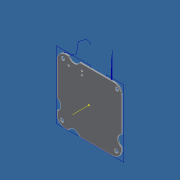
# Autodesk Inventor part: Eagle PCB
Saved by Autodesk Inventor 2016 (Build 200138000, 138)
## iProperties
Created: 2015-06-19
Part Number: Eagle PCB
Material: Generic
Document SubType Name: Modeling
Designer: Samuel Clay
Density: 1 g/cm^3
Appearance: Default
Author: Samuel Clay
Autodesk Inventor part; units mm, degrees
(part 1 of 11)
ref_plane "YZ Plane" through (0, 0, 0) normal (1, 0, 0) x (0, 1, 0)
ref_plane "XZ Plane" through (0, 0, 0) normal (0, 1, 0) x (-1, 0, 0)
ref_plane "XY Plane" through (0, 0, 0) normal (0, 0, 1) x (1, 0, 0)
sketch "1" plane through (0, 0, 0) normal (0, 0, 1) x (1, 0, 0)
  arc A0 (13.5069, 27.1331) -> (13.4171, 27.2229) centre (13.462, 27.178) ccw
  arc A1 (12.9091, 26.7149) -> (12.9989, 26.6251) centre (12.954, 26.67) ccw
  line L0 (13.462, 27.178) -> (12.954, 26.67)
  arc A2 (14.6362, 27.1145) -> (14.6362, 27.2415) centre (14.6362, 27.178) ccw
  arc A3 (13.462, 27.2415) -> (13.462, 27.1145) centre (13.462, 27.178) ccw
  line L1 (14.6362, 27.178) -> (13.462, 27.178)
  arc A4 (3.5302, 16.6256) -> (3.4404, 16.5358) centre (3.4853, 16.5807) ccw
  arc A5 (10.6231, 9.3531) -> (10.7129, 9.4429) centre (10.668, 9.398) ccw
  line L2 (3.4853, 16.5807) -> (10.668, 9.398)
  arc A6 (3.5488, 24.0433) -> (3.4218, 24.0433) centre (3.4853, 24.0433) ccw
  arc A7 (3.4218, 16.5807) -> (3.5488, 16.5807) centre (3.4853, 16.5807) ccw
  line L3 (3.4853, 24.0433) -> (3.4853, 16.5807)
  arc A8 (20.2591, 27.3871) -> (20.3489, 27.4769) centre (20.304, 27.432) ccw
  arc A9 (17.5549, 30.2709) -> (17.4651, 30.1811) centre (17.51, 30.226) ccw
  line L4 (20.304, 27.432) -> (17.51, 30.226)
  arc A10 (26.162, 27.3685) -> (26.162, 27.4955) centre (26.162, 27.432) ccw
  arc A11 (20.304, 27.4955) -> (20.304, 27.3685) centre (20.304, 27.432) ccw
  line L5 (26.162, 27.432) -> (20.304, 27.432)
  arc A12 (17.5549, 30.0069) -> (17.4651, 30.0967) centre (17.51, 30.0518) ccw
  arc A13 (15.3142, 27.9458) -> (15.404, 27.856) centre (15.3591, 27.9009) ccw
  line L6 (17.51, 30.0518) -> (15.3591, 27.9009)
  arc A14 (17.5735, 30.226) -> (17.4465, 30.226) centre (17.51, 30.226) ccw
  arc A15 (17.4465, 30.0518) -> (17.5735, 30.0518) centre (17.51, 30.0518) ccw
  line L7 (17.51, 30.226) -> (17.51, 30.0518)
  arc A16 (17.5735, 35.052) -> (17.4465, 35.052) centre (17.51, 35.052) ccw
  arc A17 (17.4465, 30.226) -> (17.5735, 30.226) centre (17.51, 30.226) ccw
  line L8 (17.51, 35.052) -> (17.51, 30.226)
  arc A18 (8.1889, 27.4609) -> (8.0991, 27.3711) centre (8.144, 27.416) ccw
  arc A19 (9.3531, 26.1171) -> (9.4429, 26.2069) centre (9.398, 26.162) ccw
  line L9 (8.144, 27.416) -> (9.398, 26.162)
  arc A20 (8.2075, 28.702) -> (8.0805, 28.702) centre (8.144, 28.702) ccw
  arc A21 (8.0805, 27.416) -> (8.2075, 27.416) centre (8.144, 27.416) ccw
  line L10 (8.144, 28.702) -> (8.144, 27.416)
  arc A22 (26.1171, 31.6777) -> (26.2069, 31.5879) centre (26.162, 31.6328) ccw
  arc A23 (27.4601, 32.8411) -> (27.3704, 32.9309) centre (27.4152, 32.886) ccw
  line L11 (26.162, 31.6328) -> (27.4153, 32.886)
  arc A24 (26.0985, 27.432) -> (26.2255, 27.432) centre (26.162, 27.432) ccw
  arc A25 (26.2255, 31.6328) -> (26.0985, 31.6328) centre (26.162, 31.6328) ccw
  line L12 (26.162, 27.432) -> (26.162, 31.6328)
  arc A26 (26.2069, 24.1749) -> (26.1171, 24.0851) centre (26.162, 24.13) ccw
  arc A27 (26.8791, 23.3231) -> (26.9689, 23.4129) centre (26.924, 23.368) ccw
  line L13 (26.162, 24.13) -> (26.924, 23.368)
  arc A28 (26.2255, 27.432) -> (26.0985, 27.432) centre (26.162, 27.432) ccw
  arc A29 (26.0985, 24.13) -> (26.2255, 24.13) centre (26.162, 24.13) ccw
  line L14 (26.162, 27.432) -> (26.162, 24.13)
  arc A30 (33.8827, 24.1749) -> (33.7929, 24.0851) centre (33.8378, 24.13) ccw
  arc A31 (34.8303, 23.0477) -> (34.9201, 23.1375) centre (34.8752, 23.0926) ccw
  line L15 (33.8378, 24.13) -> (34.8752, 23.0926)
  arc A32 (32.258, 24.1935) -> (32.258, 24.0665) centre (32.258, 24.13) ccw
  arc A33 (33.8378, 24.0665) -> (33.8378, 24.1935) centre (33.8378, 24.13) ccw
  line L16 (32.258, 24.13) -> (33.8378, 24.13)
  arc A34 (31.4511, 23.4129) -> (31.5409, 23.3231) centre (31.496, 23.368) ccw
  arc A35 (32.3029, 24.0851) -> (32.2131, 24.1749) centre (32.258, 24.13) ccw
  line L17 (31.496, 23.368) -> (32.258, 24.13)
  arc A36 (26.924, 23.4315) -> (26.924, 23.3045) centre (26.924, 23.368) ccw
  arc A37 (31.496, 23.3045) -> (31.496, 23.4315) centre (31.496, 23.368) ccw
  line L18 (26.924, 23.368) -> (31.496, 23.368)
  arc A38 (23.4571, 19.9909) -> (23.5469, 19.9011) centre (23.502, 19.946) ccw
  arc A39 (26.9689, 23.3231) -> (26.8791, 23.4129) centre (26.924, 23.368) ccw
  line L19 (23.502, 19.946) -> (26.924, 23.368)
  arc A40 (23.314, 20.0095) -> (23.314, 19.8825) centre (23.314, 19.946) ccw
  arc A41 (23.502, 19.8825) -> (23.502, 20.0095) centre (23.502, 19.946) ccw
  line L20 (23.314, 19.946) -> (23.502, 19.946)
  arc A42 (29.7389, 12.8851) -> (29.6491, 12.9749) centre (29.694, 12.93) ccw
  arc A43 (27.3871, 10.7129) -> (27.4769, 10.6231) centre (27.432, 10.668) ccw
  line L21 (29.694, 12.93) -> (27.432, 10.668)
  arc A44 (31.242, 12.8665) -> (31.242, 12.9935) centre (31.242, 12.93) ccw
  arc A45 (29.694, 12.9935) -> (29.694, 12.8665) centre (29.694, 12.93) ccw
  line L22 (31.242, 12.93) -> (29.694, 12.93)
  arc A46 (36.0231, 21.8549) -> (36.1129, 21.9447) centre (36.068, 21.8998) ccw
  arc A47 (34.9201, 23.1375) -> (34.8303, 23.0477) centre (34.8752, 23.0926) ccw
  line L23 (36.068, 21.8998) -> (34.8752, 23.0926)
  arc A48 (36.0045, 14.986) -> (36.1315, 14.986) centre (36.068, 14.986) ccw
  arc A49 (36.1315, 21.8998) -> (36.0045, 21.8998) centre (36.068, 21.8998) ccw
  line L24 (36.068, 14.986) -> (36.068, 21.8998)
  arc A50 (33.9671, 12.9749) -> (34.0569, 12.8851) centre (34.012, 12.93) ccw
  arc A51 (36.1129, 14.9411) -> (36.0231, 15.0309) centre (36.068, 14.986) ccw
  line L25 (34.012, 12.93) -> (36.068, 14.986)
  arc A52 (31.242, 12.9935) -> (31.242, 12.8665) centre (31.242, 12.93) ccw
  arc A53 (34.012, 12.8665) -> (34.012, 12.9935) centre (34.012, 12.93) ccw
  line L26 (31.242, 12.93) -> (34.012, 12.93)
  arc A54 (15.5549, 28.0069) -> (15.4651, 28.0967) centre (15.51, 28.0518) ccw
  arc A55 (15.3142, 27.9458) -> (15.404, 27.856) centre (15.3591, 27.9009) ccw
  line L27 (15.51, 28.0518) -> (15.3591, 27.9009)
  arc A56 (14.5913, 27.2229) -> (14.6811, 27.1331) centre (14.6362, 27.178) ccw
  arc A57 (15.404, 27.856) -> (15.3142, 27.9458) centre (15.3591, 27.9009) ccw
  line L28 (14.6362, 27.178) -> (15.3591, 27.9009)
  arc A58 (7.9362, 30.0011) -> (7.8118, 29.9749) centre (7.874, 29.988) ccw
  arc A59 (8.0818, 28.6889) -> (8.2062, 28.7151) centre (8.144, 28.702) ccw
  line L29 (7.874, 29.988) -> (8.144, 28.702)
  arc A60 (7.9375, 31.623) -> (7.8105, 31.623) centre (7.874, 31.623) ccw
  arc A61 (7.8105, 29.988) -> (7.9375, 29.988) centre (7.874, 29.988) ccw
  line L30 (7.874, 31.623) -> (7.874, 29.988)
  arc A62 (3.4404, 24.0882) -> (3.5302, 23.9984) centre (3.4853, 24.0433) ccw
  arc A63 (8.1889, 28.6571) -> (8.0991, 28.7469) centre (8.144, 28.702) ccw
  line L31 (3.4853, 24.0433) -> (8.144, 28.702)
  arc A64 (3.3727, 24.1068) -> (3.3727, 23.9798) centre (3.3727, 24.0433) ccw
  arc A65 (3.4853, 23.9798) -> (3.4853, 24.1068) centre (3.4853, 24.0433) ccw
  line L32 (3.3727, 24.0433) -> (3.4853, 24.0433)
  arc A66 (-1.8796, -1.524) -> (-1.6764, -1.524) centre (-1.778, -1.524) ccw
  arc A67 (-1.6764, 38.608) -> (-1.8796, 38.608) centre (-1.778, 38.608) ccw
  line L33 (-1.778, -1.524) -> (-1.778, 38.608)
  arc A68 (38.354, -1.6256) -> (38.354, -1.4224) centre (38.354, -1.524) ccw
  arc A69 (-1.778, -1.4224) -> (-1.778, -1.6256) centre (-1.778, -1.524) ccw
  line L34 (38.354, -1.524) -> (-1.778, -1.524)
  arc A70 (38.2016, 38.6086) -> (37.9984, 38.6074) centre (38.1, 38.608) ccw
  arc A71 (38.2524, -1.5246) -> (38.4556, -1.5234) centre (38.354, -1.524) ccw
  line L35 (38.1, 38.608) -> (38.354, -1.524)
  arc A72 (27.94, 38.7096) -> (27.94, 38.5064) centre (27.94, 38.608) ccw
  arc A73 (38.1, 38.5064) -> (38.1, 38.7096) centre (38.1, 38.608) ccw
  line L36 (27.94, 38.608) -> (38.1, 38.608)
  arc A74 (27.8384, 34.036) -> (28.0416, 34.036) centre (27.94, 34.036) ccw
  arc A75 (28.0416, 38.608) -> (27.8384, 38.608) centre (27.94, 38.608) ccw
  line L37 (27.94, 34.036) -> (27.94, 38.608)
  arc A76 (25.654, 34.1376) -> (25.654, 33.9344) centre (25.654, 34.036) ccw
  arc A77 (27.94, 33.9344) -> (27.94, 34.1376) centre (27.94, 34.036) ccw
  line L38 (25.654, 34.036) -> (27.94, 34.036)
  arc A78 (21.2642, 29.7898) -> (21.4078, 29.6462) centre (21.336, 29.718) ccw
  arc A79 (25.7258, 33.9642) -> (25.5822, 34.1078) centre (25.654, 34.036) ccw
  line L39 (21.336, 29.718) -> (25.654, 34.036)
  arc A80 (18.6104, 32.3332) -> (18.4736, 32.1828) centre (18.542, 32.258) ccw
  arc A81 (21.2676, 29.6428) -> (21.4044, 29.7932) centre (21.336, 29.718) ccw
  line L40 (18.542, 32.258) -> (21.336, 29.718)
  arc A82 (18.6436, 38.608) -> (18.4404, 38.608) centre (18.542, 38.608) ccw
  arc A83 (18.4404, 32.258) -> (18.6436, 32.258) centre (18.542, 32.258) ccw
  line L41 (18.542, 38.608) -> (18.542, 32.258)
  arc A84 (-1.778, 38.7096) -> (-1.778, 38.5064) centre (-1.778, 38.608) ccw
  arc A85 (18.542, 38.5064) -> (18.542, 38.7096) centre (18.542, 38.608) ccw
  line L42 (-1.778, 38.608) -> (18.542, 38.608)
  arc A86 (16.256, 16.4465) -> (16.256, 16.5735) centre (16.256, 16.51) ccw
  arc A87 (14.732, 16.5735) -> (14.732, 16.4465) centre (14.732, 16.51) ccw
  line L43 (16.256, 16.51) -> (14.732, 16.51)
  arc A88 (21.5046, 21.6688) -> (21.4148, 21.7586) centre (21.4597, 21.7137) ccw
  arc A89 (16.2111, 16.5549) -> (16.3009, 16.4651) centre (16.256, 16.51) ccw
  line L44 (21.4597, 21.7137) -> (16.256, 16.51)
  arc A90 (21.5463, 21.6502) -> (21.5463, 21.7772) centre (21.5463, 21.7137) ccw
  arc A91 (21.4597, 21.7772) -> (21.4597, 21.6503) centre (21.4597, 21.7137) ccw
  line L45 (21.5463, 21.7137) -> (21.4597, 21.7137)
  arc A92 (34.5889, 16.4651) -> (34.4991, 16.5549) centre (34.544, 16.51) ccw
  arc A93 (34.2451, 16.3009) -> (34.3349, 16.2111) centre (34.29, 16.256) ccw
  line L46 (34.544, 16.51) -> (34.29, 16.256)
  arc A94 (34.6075, 19.812) -> (34.4805, 19.812) centre (34.544, 19.812) ccw
  arc A95 (34.4805, 16.51) -> (34.6075, 16.51) centre (34.544, 16.51) ccw
  line L47 (34.544, 19.812) -> (34.544, 16.51)
  arc A96 (33.1524, 21.2934) -> (33.0626, 21.2036) centre (33.1075, 21.2485) ccw
  arc A97 (34.4991, 19.7671) -> (34.5889, 19.8569) centre (34.544, 19.812) ccw
  line L48 (33.1075, 21.2485) -> (34.544, 19.812)
  arc A98 (33.171, 21.3248) -> (33.044, 21.3248) centre (33.1075, 21.3248) ccw
  arc A99 (33.044, 21.2485) -> (33.171, 21.2485) centre (33.1075, 21.2485) ccw
  line L49 (33.1075, 21.3248) -> (33.1075, 21.2485)
  arc A100 (35.7691, 27.8951) -> (35.8589, 27.9849) centre (35.814, 27.94) ccw
  arc A101 (35.6049, 28.2389) -> (35.5151, 28.1491) centre (35.56, 28.194) ccw
  line L50 (35.814, 27.94) -> (35.56, 28.194)
  arc A102 (35.7505, 27.432) -> (35.8775, 27.432) centre (35.814, 27.432) ccw
  arc A103 (35.8775, 27.94) -> (35.7505, 27.94) centre (35.814, 27.94) ccw
  line L51 (35.814, 27.432) -> (35.814, 27.94)
  arc A104 (34.4414, 26.1492) -> (34.5312, 26.0594) centre (34.4863, 26.1043) ccw
  arc A105 (35.8589, 27.3871) -> (35.7691, 27.4769) centre (35.814, 27.432) ccw
  line L52 (34.4863, 26.1043) -> (35.814, 27.432)
  arc A106 (34.4228, 25.815) -> (34.5498, 25.815) centre (34.4863, 25.815) ccw
  arc A107 (34.5498, 26.1043) -> (34.4228, 26.1043) centre (34.4863, 26.1043) ccw
  line L53 (34.4863, 25.815) -> (34.4863, 26.1043)
  arc A108 (21.1269, 15.7031) -> (21.0371, 15.7929) centre (21.082, 15.748) ccw
  arc A109 (20.7831, 15.5389) -> (20.8729, 15.4491) centre (20.828, 15.494) ccw
  line L54 (21.082, 15.748) -> (20.828, 15.494)
  arc A110 (24.384, 15.6845) -> (24.384, 15.8115) centre (24.384, 15.748) ccw
  arc A111 (21.082, 15.8115) -> (21.082, 15.6845) centre (21.082, 15.748) ccw
  line L55 (24.384, 15.748) -> (21.082, 15.748)
  arc A112 (25.9752, 17.2494) -> (25.8854, 17.3392) centre (25.9303, 17.2943) ccw
  arc A113 (24.3391, 15.7929) -> (24.4289, 15.7031) centre (24.384, 15.748) ccw
  line L56 (25.9303, 17.2943) -> (24.384, 15.748)
  arc A114 (25.9657, 17.2308) -> (25.9657, 17.3578) centre (25.9657, 17.2943) ccw
  arc A115 (25.9303, 17.3578) -> (25.9303, 17.2308) centre (25.9303, 17.2943) ccw
  line L57 (25.9657, 17.2943) -> (25.9303, 17.2943)
  arc A116 (30.022, 30.3658) -> (30.1118, 30.276) centre (30.0669, 30.3209) ccw
  arc A117 (32.5569, 32.7211) -> (32.4671, 32.8109) centre (32.512, 32.766) ccw
  line L58 (30.0669, 30.3209) -> (32.512, 32.766)
  arc A118 (30.0034, 30.2344) -> (30.1304, 30.2344) centre (30.0669, 30.2344) ccw
  arc A119 (30.1304, 30.3209) -> (30.0034, 30.3209) centre (30.0669, 30.3209) ccw
  line L59 (30.0669, 30.2344) -> (30.0669, 30.3209)
  arc A120 (9.3345, 19.304) -> (9.4615, 19.304) centre (9.398, 19.304) ccw
  arc A121 (9.4615, 20.32) -> (9.3345, 20.32) centre (9.398, 20.32) ccw
  line L60 (9.398, 19.304) -> (9.398, 20.32)
  arc A122 (13.9251, 14.6871) -> (14.0149, 14.7769) centre (13.97, 14.732) ccw
  arc A123 (9.4429, 19.3489) -> (9.3531, 19.2591) centre (9.398, 19.304) ccw
  line L61 (13.97, 14.732) -> (9.398, 19.304)
  arc A124 (27.432, 14.6685) -> (27.432, 14.7955) centre (27.432, 14.732) ccw
  arc A125 (13.97, 14.7955) -> (13.97, 14.6685) centre (13.97, 14.732) ccw
  line L62 (27.432, 14.732) -> (13.97, 14.732)
  arc A126 (28.7329, 15.9431) -> (28.6431, 16.0329) centre (28.688, 15.988) ccw
  arc A127 (27.3871, 14.7769) -> (27.4769, 14.6871) centre (27.432, 14.732) ccw
  line L63 (28.6881, 15.9881) -> (27.432, 14.732)
  arc A128 (28.7516, 16.9054) -> (28.6246, 16.9054) centre (28.6881, 16.9054) ccw
  arc A129 (28.6246, 15.9881) -> (28.7515, 15.9881) centre (28.6881, 15.9881) ccw
  line L64 (28.6881, 16.9054) -> (28.6881, 15.9881)
  arc A130 (29.1405, 31.2622) -> (29.2255, 31.1678) centre (29.183, 31.215) ccw
  arc A131 (31.7925, 33.4808) -> (31.7075, 33.5752) centre (31.75, 33.528) ccw
  line L65 (29.183, 31.215) -> (31.75, 33.528)
  arc A132 (29.1195, 31.1183) -> (29.2465, 31.1183) centre (29.183, 31.1183) ccw
  arc A133 (29.2465, 31.215) -> (29.1195, 31.215) centre (29.183, 31.215) ccw
  line L66 (29.183, 31.1183) -> (29.183, 31.215)
  arc A134 (31.9591, 16.3009) -> (32.0489, 16.2111) centre (32.004, 16.256) ccw
  arc A135 (33.5729, 17.7351) -> (33.4831, 17.8249) centre (33.528, 17.78) ccw
  line L67 (32.004, 16.256) -> (33.528, 17.78)
  arc A136 (31.242, 16.3195) -> (31.242, 16.1925) centre (31.242, 16.256) ccw
  arc A137 (32.004, 16.1925) -> (32.004, 16.3195) centre (32.004, 16.256) ccw
  line L68 (31.242, 16.256) -> (32.004, 16.256)
  arc A138 (29.7536, 17.8342) -> (29.6638, 17.7444) centre (29.7087, 17.7893) ccw
  arc A139 (31.1971, 16.2111) -> (31.2869, 16.3009) centre (31.242, 16.256) ccw
  line L69 (29.7087, 17.7893) -> (31.242, 16.256)
  arc A140 (29.5719, 17.8528) -> (29.5719, 17.7258) centre (29.5719, 17.7893) ccw
  arc A141 (29.7087, 17.7258) -> (29.7087, 17.8528) centre (29.7087, 17.7893) ccw
  line L70 (29.5719, 17.7893) -> (29.7087, 17.7893)
  arc A142 (12.291, 17.7883) -> (12.2011, 17.6985) centre (12.2461, 17.7434) ccw
  arc A143 (13.4265, 16.4731) -> (13.5163, 16.5629) centre (13.4714, 16.518) ccw
  line L71 (12.2461, 17.7434) -> (13.4714, 16.518)
  arc A144 (12.2656, 17.7873) -> (12.1386, 17.7873) centre (12.2021, 17.7873) ccw
  arc A145 (12.1826, 17.7434) -> (12.3096, 17.7434) centre (12.2461, 17.7434) ccw
  line L72 (12.2021, 17.7873) -> (12.2461, 17.7434)
  arc A146 (6.3949, 33.4831) -> (6.3051, 33.5729) centre (6.35, 33.528) ccw
  arc A147 (4.0191, 31.2869) -> (4.1089, 31.1971) centre (4.064, 31.242) ccw
  line L73 (6.35, 33.528) -> (4.064, 31.242)
  arc A148 (7.112, 33.4645) -> (7.112, 33.5915) centre (7.112, 33.528) ccw
  arc A149 (6.35, 33.5915) -> (6.35, 33.4645) centre (6.35, 33.528) ccw
  line L74 (7.112, 33.528) -> (6.35, 33.528)
  arc A150 (7.7021, 32.8481) -> (7.7919, 32.9379) centre (7.747, 32.893) ccw
  arc A151 (7.1569, 33.5729) -> (7.0671, 33.4831) centre (7.112, 33.528) ccw
  line L75 (7.747, 32.893) -> (7.112, 33.528)
  arc A152 (7.874, 32.8295) -> (7.874, 32.9565) centre (7.874, 32.893) ccw
  arc A153 (7.747, 32.9565) -> (7.747, 32.8295) centre (7.747, 32.893) ccw
  line L76 (7.874, 32.893) -> (7.747, 32.893)
  arc A154 (14.1627, 32.3371) -> (14.2525, 32.2473) centre (14.2076, 32.2922) ccw
  arc A155 (14.9879, 33.0349) -> (14.8981, 33.1248) centre (14.943, 33.0799) ccw
  line L77 (14.2076, 32.2922) -> (14.943, 33.0799)
  arc A156 (13.1762, 32.3203) -> (13.1762, 32.1933) centre (13.1762, 32.2568) ccw
  arc A157 (14.2076, 32.2287) -> (14.2076, 32.3557) centre (14.2076, 32.2922) ccw
  line L78 (13.1762, 32.2568) -> (14.2076, 32.2922)
  arc A158 (12.5185, 31.6452) -> (12.6083, 31.5554) centre (12.5634, 31.6003) ccw
  arc A159 (13.2211, 32.2119) -> (13.1313, 32.3017) centre (13.1762, 32.2568) ccw
  line L79 (12.5634, 31.6003) -> (13.1762, 32.2568)
  arc A160 (12.4364, 31.6595) -> (12.4364, 31.5325) centre (12.4364, 31.596) ccw
  arc A161 (12.5634, 31.5368) -> (12.5634, 31.6638) centre (12.5634, 31.6003) ccw
  line L80 (12.4364, 31.596) -> (12.5634, 31.6003)
  arc A162 (13.7799, 25.2104) -> (13.8639, 25.1151) centre (13.8219, 25.1627) ccw
  arc A163 (15.9235, 27.0579) -> (15.8395, 27.1532) centre (15.8815, 27.1056) ccw
  line L81 (13.8219, 25.1627) -> (15.8815, 27.1056)
  arc A164 (12.9125, 25.195) -> (12.9125, 25.068) centre (12.9125, 25.1315) ccw
  arc A165 (13.8219, 25.0992) -> (13.8219, 25.2262) centre (13.8219, 25.1627) ccw
  line L82 (12.9125, 25.1315) -> (13.8219, 25.1627)
  arc A166 (11.8288, 26.2301) -> (11.739, 26.1403) centre (11.7839, 26.1852) ccw
  arc A167 (11.6996, 27.3767) -> (11.7894, 27.287) centre (11.7445, 27.3318) ccw
  line L83 (13.0154, 28.6931) -> (11.7445, 27.3318)
  arc A168 (14.5675, 28.6829) -> (14.5675, 28.8099) centre (14.5675, 28.7464) ccw
  arc A169 (13.0154, 28.7566) -> (13.0154, 28.6296) centre (13.0154, 28.6931) ccw
  line L84 (14.5675, 28.7464) -> (13.0154, 28.6931)
  arc A170 (15.7365, 29.9056) -> (15.6467, 29.9954) centre (15.6916, 29.9505) ccw
  arc A171 (14.5226, 28.7913) -> (14.6124, 28.7015) centre (14.5675, 28.7464) ccw
  line L85 (15.6916, 29.9505) -> (14.5675, 28.7464)
  arc A172 (15.7305, 30.6685) -> (15.6035, 30.6685) centre (15.667, 30.6685) ccw
  arc A173 (15.6281, 29.9505) -> (15.7551, 29.9505) centre (15.6916, 29.9505) ccw
  line L86 (15.667, 30.6685) -> (15.6916, 29.9505)
  arc A174 (15.0495, 31.3318) -> (14.9597, 31.242) centre (15.0046, 31.2869) ccw
  arc A175 (15.6221, 30.6236) -> (15.7119, 30.7134) centre (15.667, 30.6685) ccw
  line L87 (15.0046, 31.2869) -> (15.667, 30.6685)
  arc A176 (15.0065, 33.0799) -> (14.8795, 33.0799) centre (14.943, 33.0799) ccw
  arc A177 (14.9411, 31.2869) -> (15.0681, 31.2869) centre (15.0046, 31.2869) ccw
  line L88 (14.943, 33.0799) -> (15.0046, 31.2869)
  arc A178 (14.9368, 35.1107) -> (14.8098, 35.1107) centre (14.8733, 35.1107) ccw
  arc A179 (14.8795, 33.0799) -> (15.0065, 33.0799) centre (14.943, 33.0799) ccw
  line L89 (14.8733, 35.1107) -> (14.943, 33.0799)
  arc A180 (13.5178, 16.5614) -> (13.425, 16.4747) centre (13.4714, 16.518) ccw
  arc A181 (13.6788, 16.2208) -> (13.7717, 16.3075) centre (13.7252, 16.2642) ccw
  line L90 (13.4714, 16.518) -> (13.7252, 16.2642)
  arc A182 (12.2486, 17.8306) -> (12.1557, 17.7439) centre (12.2021, 17.7873) ccw
  arc A183 (13.425, 16.4747) -> (13.5178, 16.5614) centre (13.4714, 16.518) ccw
  line L91 (12.2021, 17.7873) -> (13.4714, 16.518)
  arc A184 (10.0705, 20.0087) -> (9.9777, 19.922) centre (10.0241, 19.9654) ccw
  arc A185 (12.1557, 17.7439) -> (12.2486, 17.8306) centre (12.2021, 17.7873) ccw
  line L92 (10.0241, 19.9654) -> (12.2021, 17.7873)
  arc A186 (9.7918, 28.5803) -> (9.6648, 28.5803) centre (9.7283, 28.5803) ccw
  arc A187 (9.9606, 19.9654) -> (10.0876, 19.9654) centre (10.0241, 19.9654) ccw
  line L93 (9.7283, 28.5803) -> (10.0241, 19.9654)
  arc A188 (15.746, 15.3634) -> (15.8358, 15.2736) centre (15.7909, 15.3185) ccw
  arc A189 (16.0825, 15.5377) -> (15.9911, 15.626) centre (16.036, 15.5811) ccw
  line L94 (15.7909, 15.3185) -> (16.036, 15.5811)
  arc A190 (14.7755, 15.3471) -> (14.7755, 15.2201) centre (14.7755, 15.2836) ccw
  arc A191 (15.7909, 15.255) -> (15.7909, 15.382) centre (15.7909, 15.3185) ccw
  line L95 (14.7755, 15.2836) -> (15.7909, 15.3185)
  arc A192 (13.7701, 16.3091) -> (13.6803, 16.2193) centre (13.7252, 16.2642) ccw
  arc A193 (14.7306, 15.2387) -> (14.8204, 15.3285) centre (14.7755, 15.2836) ccw
  line L96 (13.7252, 16.2642) -> (14.7755, 15.2836)
  arc A194 (13.5709, 22.6104) -> (13.4439, 22.6104) centre (13.5074, 22.6104) ccw
  arc A195 (13.6617, 16.2642) -> (13.7887, 16.2642) centre (13.7252, 16.2642) ccw
  line L97 (13.5074, 22.6104) -> (13.7252, 16.2642)
  arc A196 (16.8441, 26.0914) -> (16.7543, 26.1812) centre (16.7992, 26.1363) ccw
  arc A197 (13.4625, 22.6553) -> (13.5523, 22.5655) centre (13.5074, 22.6104) ccw
  line L98 (16.7992, 26.1363) -> (13.5074, 22.6104)
  arc A198 (16.8587, 26.2525) -> (16.7317, 26.2525) centre (16.7952, 26.2525) ccw
  arc A199 (16.7357, 26.1363) -> (16.8627, 26.1363) centre (16.7992, 26.1363) ccw
  line L99 (16.7952, 26.2525) -> (16.7992, 26.1363)
  line L100 (17.78, 13.208) -> (17.78, 9.636)
  arc A200 (16.2537, 15.291) -> (16.3435, 15.3808) centre (16.2986, 15.3359) ccw
  arc A201 (16.0809, 15.626) -> (15.9927, 15.5346) centre (16.036, 15.5811) ccw
  line L101 (16.2986, 15.3359) -> (16.036, 15.5811)
  arc A202 (16.8063, 15.2898) -> (16.8063, 15.4168) centre (16.8063, 15.3533) ccw
  arc A203 (16.2986, 15.3994) -> (16.2986, 15.2724) centre (16.2986, 15.3359) ccw
  line L102 (16.8063, 15.3533) -> (16.2986, 15.3359)
  arc A204 (22.246, 21.0868) -> (22.1562, 21.1766) centre (22.2011, 21.1317) ccw
  arc A205 (16.7614, 15.3982) -> (16.8512, 15.3084) centre (16.8063, 15.3533) ccw
  line L103 (22.2011, 21.1317) -> (16.8063, 15.3533)
  arc A206 (22.2773, 21.0708) -> (22.2773, 21.1978) centre (22.2773, 21.1343) ccw
  arc A207 (22.2011, 21.1952) -> (22.2011, 21.0682) centre (22.2011, 21.1317) ccw
  line L104 (22.2773, 21.1343) -> (22.2011, 21.1317)
  arc A208 (35.2611, 20.8492) -> (35.3509, 20.939) centre (35.306, 20.8941) ccw
  arc A209 (34.0363, 22.2536) -> (33.9464, 22.1638) centre (33.9913, 22.2087) ccw
  line L105 (35.306, 20.8941) -> (33.9913, 22.2087)
  arc A210 (35.2425, 15.494) -> (35.3695, 15.494) centre (35.306, 15.494) ccw
  arc A211 (35.3695, 20.8941) -> (35.2425, 20.8941) centre (35.306, 20.8941) ccw
  line L106 (35.306, 15.494) -> (35.306, 20.8941)
  arc A212 (33.9911, 14.2689) -> (34.0809, 14.1791) centre (34.036, 14.224) ccw
  arc A213 (35.3509, 15.4491) -> (35.2611, 15.5389) centre (35.306, 15.494) ccw
  line L107 (34.036, 14.224) -> (35.306, 15.494)
  arc A214 (29.718, 14.2875) -> (29.718, 14.1605) centre (29.718, 14.224) ccw
  arc A215 (34.036, 14.1605) -> (34.036, 14.2875) centre (34.036, 14.224) ccw
  line L108 (29.718, 14.224) -> (34.036, 14.224)
  arc A216 (26.1171, 10.7129) -> (26.2069, 10.6231) centre (26.162, 10.668) ccw
  arc A217 (29.7629, 14.1791) -> (29.6731, 14.2689) centre (29.718, 14.224) ccw
  line L109 (26.162, 10.668) -> (29.718, 14.224)
  arc A218 (26.0985, 9.652) -> (26.2255, 9.652) centre (26.162, 9.652) ccw
  arc A219 (26.2255, 10.668) -> (26.0985, 10.668) centre (26.162, 10.668) ccw
  line L110 (26.162, 9.652) -> (26.162, 10.668)
  arc A220 (26.6251, 9.0991) -> (26.7149, 9.1889) centre (26.67, 9.144) ccw
  arc A221 (26.2069, 9.6969) -> (26.1171, 9.6071) centre (26.162, 9.652) ccw
  line L111 (26.67, 9.144) -> (26.162, 9.652)
  arc A222 (27.432, 9.0805) -> (27.432, 9.2075) centre (27.432, 9.144) ccw
  arc A223 (26.67, 9.2075) -> (26.67, 9.0805) centre (26.67, 9.144) ccw
  line L112 (27.432, 9.144) -> (26.67, 9.144)
  arc A224 (28.2629, 9.8851) -> (28.1731, 9.9749) centre (28.218, 9.93) ccw
  arc A225 (27.3871, 9.1889) -> (27.4769, 9.0991) centre (27.432, 9.144) ccw
  line L113 (28.218, 9.93) -> (27.432, 9.144)
  arc A226 (31.242, 9.8665) -> (31.242, 9.9935) centre (31.242, 9.93) ccw
  arc A227 (28.218, 9.9935) -> (28.218, 9.8665) centre (28.218, 9.93) ccw
  line L114 (31.242, 9.93) -> (28.218, 9.93)
  arc A228 (30.6135, 9.8851) -> (30.5237, 9.9749) centre (30.5686, 9.93) ccw
  arc A229 (23.9824, 3.4336) -> (24.0722, 3.3438) centre (24.0273, 3.3887) ccw
  arc A230 (15.9264, 27.1505) -> (15.8366, 27.0607) centre (15.8815, 27.1056) ccw
  line L115 (30.5686, 9.93) -> (24.0273, 3.3887)
  arc A231 (31.242, 9.8665) -> (31.242, 9.9935) centre (31.242, 9.93) ccw
  arc A232 (30.5686, 9.9935) -> (30.5686, 9.8665) centre (30.5686, 9.93) ccw
  line L116 (31.242, 9.93) -> (30.5686, 9.93)
  arc A233 (16.7503, 26.2076) -> (16.8401, 26.2974) centre (16.7952, 26.2525) ccw
  line L117 (15.8815, 27.1056) -> (16.7952, 26.2525)
  arc A234 (17.8249, 9.6809) -> (17.7351, 9.5911) centre (17.78, 9.636) ccw
  arc A235 (23.9824, 3.3438) -> (24.0722, 3.4336) centre (24.0273, 3.3887) ccw
  line L118 (17.78, 9.636) -> (24.0273, 3.3887)
  arc A236 (17.8435, 13.208) -> (17.7165, 13.208) centre (17.78, 13.208) ccw
  arc A237 (17.7165, 9.636) -> (17.8435, 9.636) centre (17.78, 9.636) ccw
  arc A238 (12.8676, 25.0866) -> (12.9574, 25.1764) centre (12.9125, 25.1315) ccw
  line L119 (11.7839, 26.1852) -> (12.9125, 25.1315)
  arc A239 (11.808, 27.3318) -> (11.681, 27.3318) centre (11.7445, 27.3318) ccw
  arc A240 (11.7204, 26.1852) -> (11.8474, 26.1852) centre (11.7839, 26.1852) ccw
  line L120 (11.7445, 27.3318) -> (11.7839, 26.1852)
  arc A241 (13.0603, 28.6482) -> (12.9705, 28.738) centre (13.0154, 28.6931) ccw
  arc A242 (11.6205, 30.734) -> (11.7475, 30.734) centre (11.684, 30.734) ccw
  arc A243 (11.7475, 31.623) -> (11.6205, 31.623) centre (11.684, 31.623) ccw
  line L121 (11.684, 30.734) -> (11.684, 31.623)
  arc A244 (12.1471, 30.1811) -> (12.2369, 30.2709) centre (12.192, 30.226) ccw
  arc A245 (11.7289, 30.7789) -> (11.6391, 30.6891) centre (11.684, 30.734) ccw
  line L122 (12.192, 30.226) -> (11.684, 30.734)
  arc A246 (15.494, 30.1625) -> (15.494, 30.2895) centre (15.494, 30.226) ccw
  arc A247 (12.192, 30.2895) -> (12.192, 30.1625) centre (12.192, 30.226) ccw
  line L123 (15.494, 30.226) -> (12.192, 30.226)
  arc A248 (28.2591, 32.1585) -> (28.3391, 32.0598) centre (28.2991, 32.1091) ccw
  arc A249 (31.028, 34.2407) -> (30.948, 34.3393) centre (30.988, 34.29) ccw
  line L124 (28.2991, 32.1091) -> (30.988, 34.29)
  arc A250 (28.2356, 32.0021) -> (28.3626, 32.0021) centre (28.2991, 32.0021) ccw
  arc A251 (28.3626, 32.1091) -> (28.2356, 32.1091) centre (28.2991, 32.1091) ccw
  line L125 (28.2991, 32.0021) -> (28.2991, 32.1091)
  arc A252 (11.2395, 27.432) -> (11.1125, 27.432) centre (11.176, 27.432) ccw
  arc A253 (11.1125, 20.32) -> (11.2395, 20.32) centre (11.176, 20.32) ccw
  line L126 (11.176, 27.432) -> (11.176, 20.32)
  arc A254 (11.7289, 27.8951) -> (11.6391, 27.9849) centre (11.684, 27.94) ccw
  arc A255 (11.1311, 27.4769) -> (11.2209, 27.3871) centre (11.176, 27.432) ccw
  line L127 (11.684, 27.94) -> (11.176, 27.432)
  arc A256 (11.7475, 29.464) -> (11.6205, 29.464) centre (11.684, 29.464) ccw
  arc A257 (11.6205, 27.94) -> (11.7475, 27.94) centre (11.684, 27.94) ccw
  line L128 (11.684, 29.464) -> (11.684, 27.94)
  arc A258 (10.9669, 30.2709) -> (10.8771, 30.1811) centre (10.922, 30.226) ccw
  arc A259 (11.6391, 29.4191) -> (11.7289, 29.5089) centre (11.684, 29.464) ccw
  line L129 (10.922, 30.226) -> (11.684, 29.464)
  arc A260 (9.652, 30.2895) -> (9.652, 30.1625) centre (9.652, 30.226) ccw
  arc A261 (10.922, 30.1625) -> (10.922, 30.2895) centre (10.922, 30.226) ccw
  line L130 (9.652, 30.226) -> (10.922, 30.226)
  arc A262 (9.1889, 30.7789) -> (9.0991, 30.6891) centre (9.144, 30.734) ccw
  arc A263 (9.6071, 30.1811) -> (9.6969, 30.2709) centre (9.652, 30.226) ccw
  line L131 (9.144, 30.734) -> (9.652, 30.226)
  arc A264 (9.2075, 31.623) -> (9.0805, 31.623) centre (9.144, 31.623) ccw
  arc A265 (9.0805, 30.734) -> (9.2075, 30.734) centre (9.144, 30.734) ccw
  line L132 (9.144, 31.623) -> (9.144, 30.734)
  arc A266 (18.0556, 25.0778) -> (17.9658, 25.1676) centre (18.0107, 25.1227) ccw
  arc A267 (14.9411, 22.1429) -> (15.0309, 22.0531) centre (14.986, 22.098) ccw
  line L133 (18.0107, 25.1227) -> (14.986, 22.098)
  arc A268 (18.0742, 25.2493) -> (17.9472, 25.2493) centre (18.0107, 25.2493) ccw
  arc A269 (17.9472, 25.1227) -> (18.0742, 25.1227) centre (18.0107, 25.1227) ccw
  line L134 (18.0107, 25.2493) -> (18.0107, 25.1227)
  arc A270 (16.9731, 22.5337) -> (17.0629, 22.4439) centre (17.018, 22.4888) ccw
  arc A271 (18.9395, 24.3205) -> (18.8497, 24.4103) centre (18.8946, 24.3654) ccw
  line L135 (17.018, 22.4888) -> (18.8946, 24.3654)
  arc A272 (16.9545, 22.352) -> (17.0815, 22.352) centre (17.018, 22.352) ccw
  arc A273 (17.0815, 22.4888) -> (16.9545, 22.4888) centre (17.018, 22.4888) ccw
  line L136 (17.018, 22.352) -> (17.018, 22.4888)
  arc A274 (6.3949, 34.7531) -> (6.3051, 34.8429) centre (6.35, 34.798) ccw
  arc A275 (5.5431, 34.0809) -> (5.6329, 33.9911) centre (5.588, 34.036) ccw
  line L137 (6.35, 34.798) -> (5.588, 34.036)
  arc A276 (7.112, 34.7345) -> (7.112, 34.8615) centre (7.112, 34.798) ccw
  arc A277 (6.35, 34.8615) -> (6.35, 34.7345) centre (6.35, 34.798) ccw
  line L138 (7.112, 34.798) -> (6.35, 34.798)
  arc A278 (8.9721, 32.8481) -> (9.0619, 32.9379) centre (9.017, 32.893) ccw
  arc A279 (7.1569, 34.8429) -> (7.0671, 34.7531) centre (7.112, 34.798) ccw
  line L139 (9.017, 32.893) -> (7.112, 34.798)
  arc A280 (9.144, 32.8295) -> (9.144, 32.9565) centre (9.144, 32.893) ccw
  arc A281 (9.017, 32.9565) -> (9.017, 32.8295) centre (9.017, 32.893) ccw
  line L140 (9.144, 32.893) -> (9.017, 32.893)
  constraints: 778 point on circle, 282 centre point, 282 end point, 40 point on line
sketch "16" plane through (0, 0, 0) normal (0, 0, 1) x (1, 0, 0)
  arc A0 (25.6225, 22.4288) -> (25.6171, 22.3528) centre (25.6198, 22.3908) ccw
  arc A1 (15.3606, 8.8011) -> (15.3606, 8.8773) centre (15.3606, 8.8392) ccw
  arc A2 (14.0591, 8.8773) -> (14.0591, 8.8011) centre (14.0591, 8.8392) ccw
  line L0 (5.9643, 8.6868) -> (7.381, 8.6868)
  arc A3 (7.381, 8.6487) -> (7.381, 8.7249) centre (7.381, 8.6868) ccw
  arc A4 (5.9643, 8.7249) -> (5.9643, 8.6487) centre (5.9643, 8.6868) ccw
  line L1 (13.9689, 8.6868) -> (15.2977, 8.6868)
  arc A5 (15.2977, 8.6487) -> (15.2977, 8.7249) centre (15.2977, 8.6868) ccw
  arc A6 (13.9689, 8.7249) -> (13.9689, 8.6487) centre (13.9689, 8.6868) ccw
  line L2 (6.0361, 8.5344) -> (7.4777, 8.5344)
  arc A7 (7.4777, 8.4963) -> (7.4777, 8.5725) centre (7.4777, 8.5344) ccw
  arc A8 (6.0361, 8.5725) -> (6.0361, 8.4963) centre (6.0361, 8.5344) ccw
  line L3 (13.8788, 8.5344) -> (15.2204, 8.5344)
  arc A9 (15.2204, 8.4963) -> (15.2204, 8.5725) centre (15.2204, 8.5344) ccw
  arc A10 (13.8788, 8.5725) -> (13.8788, 8.4963) centre (13.8788, 8.5344) ccw
  line L4 (6.1079, 8.382) -> (7.5748, 8.382)
  arc A11 (7.5748, 8.3439) -> (7.5748, 8.4201) centre (7.5748, 8.382) ccw
  arc A12 (6.1079, 8.4201) -> (6.1079, 8.3439) centre (6.1079, 8.382) ccw
  line L5 (13.7757, 8.382) -> (15.1433, 8.382)
  arc A13 (15.1433, 8.3439) -> (15.1433, 8.4201) centre (15.1433, 8.382) ccw
  arc A14 (13.7757, 8.4201) -> (13.7757, 8.3439) centre (13.7757, 8.382) ccw
  line L6 (6.1797, 8.2296) -> (7.7021, 8.2296)
  arc A15 (7.7021, 8.1915) -> (7.7021, 8.2677) centre (7.7021, 8.2296) ccw
  arc A16 (6.1797, 8.2677) -> (6.1797, 8.1915) centre (6.1797, 8.2296) ccw
  line L7 (13.6531, 8.2296) -> (15.0661, 8.2296)
  arc A17 (15.0661, 8.1915) -> (15.0661, 8.2677) centre (15.0661, 8.2296) ccw
  arc A18 (13.6531, 8.2677) -> (13.6531, 8.1915) centre (13.6531, 8.2296) ccw
  line L8 (6.2658, 8.0772) -> (7.8295, 8.0772)
  arc A19 (7.8295, 8.0391) -> (7.8295, 8.1153) centre (7.8295, 8.0772) ccw
  arc A20 (6.2658, 8.1153) -> (6.2658, 8.0391) centre (6.2658, 8.0772) ccw
  line L9 (13.5306, 8.0772) -> (14.9755, 8.0772)
  arc A21 (14.9755, 8.0391) -> (14.9755, 8.1153) centre (14.9755, 8.0772) ccw
  arc A22 (13.5306, 8.1153) -> (13.5306, 8.0391) centre (13.5306, 8.0772) ccw
  line L10 (6.3637, 7.9248) -> (7.9784, 7.9248)
  arc A23 (7.9784, 7.8867) -> (7.9784, 7.9629) centre (7.9784, 7.9248) ccw
  arc A24 (6.3637, 7.9629) -> (6.3637, 7.8867) centre (6.3637, 7.9248) ccw
  line L11 (13.3791, 7.9248) -> (14.8723, 7.9248)
  arc A25 (14.8723, 7.8867) -> (14.8723, 7.9629) centre (14.8723, 7.9248) ccw
  arc A26 (13.3791, 7.9629) -> (13.3791, 7.8867) centre (13.3791, 7.9248) ccw
  line L12 (6.4617, 7.7724) -> (8.144, 7.7724)
  arc A27 (8.144, 7.7343) -> (8.144, 7.8105) centre (8.144, 7.7724) ccw
  arc A28 (6.4617, 7.8105) -> (6.4617, 7.7343) centre (6.4617, 7.7724) ccw
  line L13 (13.2159, 7.7724) -> (14.769, 7.7724)
  arc A29 (14.769, 7.7343) -> (14.769, 7.8105) centre (14.769, 7.7724) ccw
  arc A30 (13.2159, 7.8105) -> (13.2159, 7.7343) centre (13.2159, 7.7724) ccw
  line L14 (6.5596, 7.62) -> (8.3301, 7.62)
  arc A31 (8.3301, 7.5819) -> (8.3301, 7.6581) centre (8.3301, 7.62) ccw
  arc A32 (6.5596, 7.6581) -> (6.5596, 7.5819) centre (6.5596, 7.62) ccw
  line L15 (13.0327, 7.62) -> (14.6658, 7.62)
  arc A33 (14.6658, 7.5819) -> (14.6658, 7.6581) centre (14.6658, 7.62) ccw
  arc A34 (13.0327, 7.6581) -> (13.0327, 7.5819) centre (13.0327, 7.62) ccw
  line L16 (6.6868, 7.4676) -> (8.5468, 7.4676)
  arc A35 (8.5468, 7.4295) -> (8.5468, 7.5057) centre (8.5468, 7.4676) ccw
  arc A36 (6.6868, 7.5057) -> (6.6868, 7.4295) centre (6.6868, 7.4676) ccw
  line L17 (12.8138, 7.4676) -> (14.5337, 7.4676)
  arc A37 (14.5337, 7.4295) -> (14.5337, 7.5057) centre (14.5337, 7.4676) ccw
  arc A38 (12.8138, 7.5057) -> (12.8138, 7.4295) centre (12.8138, 7.4676) ccw
  line L18 (6.8157, 7.3152) -> (8.8055, 7.3152)
  arc A39 (8.8055, 7.2771) -> (8.8055, 7.3533) centre (8.8055, 7.3152) ccw
  arc A40 (6.8157, 7.3533) -> (6.8157, 7.2771) centre (6.8157, 7.3152) ccw
  line L19 (12.5622, 7.3152) -> (14.3995, 7.3152)
  arc A41 (14.3995, 7.2771) -> (14.3995, 7.3533) centre (14.3995, 7.3152) ccw
  arc A42 (12.5622, 7.3533) -> (12.5622, 7.2771) centre (12.5622, 7.3152) ccw
  line L20 (6.9446, 7.1628) -> (9.0876, 7.2084)
  arc A43 (9.0876, 7.1703) -> (9.0876, 7.2465) centre (9.0876, 7.2084) ccw
  arc A44 (6.9446, 7.2009) -> (6.9446, 7.1247) centre (6.9446, 7.1628) ccw
  line L21 (12.2587, 7.1628) -> (14.2653, 7.1628)
  arc A45 (14.2653, 7.1247) -> (14.2653, 7.2009) centre (14.2653, 7.1628) ccw
  arc A46 (12.2587, 7.2009) -> (12.2587, 7.1247) centre (12.2587, 7.1628) ccw
  line L22 (7.0995, 7.0104) -> (9.2669, 7.6136)
  arc A47 (9.2669, 7.5755) -> (9.2669, 7.6517) centre (9.2669, 7.6136) ccw
  arc A48 (7.0995, 7.0485) -> (7.0995, 6.9723) centre (7.0995, 7.0104) ccw
  line L23 (11.8274, 7.0104) -> (14.1047, 7.0104)
  arc A49 (14.1047, 6.9723) -> (14.1047, 7.0485) centre (14.1047, 7.0104) ccw
  arc A50 (11.8274, 7.0485) -> (11.8274, 6.9723) centre (11.8274, 7.0104) ccw
  line L24 (7.2672, 6.858) -> (10.4902, 6.858)
  arc A51 (10.4902, 6.8199) -> (10.4902, 6.8961) centre (10.4902, 6.858) ccw
  arc A52 (7.2672, 6.8961) -> (7.2672, 6.8199) centre (7.2672, 6.858) ccw
  line L25 (10.668, 6.858) -> (13.9317, 6.858)
  arc A53 (13.9317, 6.8199) -> (13.9317, 6.8961) centre (13.9317, 6.858) ccw
  arc A54 (10.668, 6.8961) -> (10.668, 6.8199) centre (10.668, 6.858) ccw
  line L26 (7.4349, 6.7056) -> (10.4902, 6.7056)
  arc A55 (10.4902, 6.6675) -> (10.4902, 6.7437) centre (10.4902, 6.7056) ccw
  arc A56 (7.4349, 6.7437) -> (7.4349, 6.6675) centre (7.4349, 6.7056) ccw
  line L27 (10.668, 6.7056) -> (13.7586, 6.7056)
  arc A57 (13.7586, 6.6675) -> (13.7586, 6.7437) centre (13.7586, 6.7056) ccw
  arc A58 (10.668, 6.7437) -> (10.668, 6.6675) centre (10.668, 6.7056) ccw
  line L28 (7.6435, 6.5532) -> (10.4902, 6.5532)
  arc A59 (10.4902, 6.5151) -> (10.4902, 6.5913) centre (10.4902, 6.5532) ccw
  arc A60 (7.6435, 6.5913) -> (7.6435, 6.5151) centre (7.6435, 6.5532) ccw
  line L29 (10.668, 6.5533) -> (13.5432, 6.5532)
  arc A61 (13.5432, 6.5151) -> (13.5432, 6.5913) centre (13.5432, 6.5532) ccw
  arc A62 (10.668, 6.5914) -> (10.668, 6.5152) centre (10.668, 6.5533) ccw
  line L30 (7.863, 6.4008) -> (10.4902, 6.4008)
  arc A63 (10.4902, 6.3627) -> (10.4902, 6.4389) centre (10.4902, 6.4008) ccw
  arc A64 (7.863, 6.4389) -> (7.863, 6.3627) centre (7.863, 6.4008) ccw
  line L31 (10.668, 6.4009) -> (13.3183, 6.4008)
  arc A65 (13.3183, 6.3627) -> (13.3183, 6.4389) centre (13.3183, 6.4008) ccw
  arc A66 (10.668, 6.439) -> (10.668, 6.3628) centre (10.668, 6.4009) ccw
  line L32 (8.1088, 6.2484) -> (10.4902, 6.2484)
  arc A67 (10.4902, 6.2103) -> (10.4902, 6.2865) centre (10.4902, 6.2484) ccw
  arc A68 (8.1088, 6.2865) -> (8.1088, 6.2103) centre (8.1088, 6.2484) ccw
  line L33 (10.668, 6.2484) -> (13.0639, 6.2484)
  arc A69 (13.0639, 6.2103) -> (13.0639, 6.2865) centre (13.0639, 6.2484) ccw
  arc A70 (10.668, 6.2865) -> (10.668, 6.2103) centre (10.668, 6.2484) ccw
  line L34 (8.4045, 6.096) -> (10.4902, 6.096)
  arc A71 (10.4902, 6.0579) -> (10.4902, 6.1341) centre (10.4902, 6.096) ccw
  arc A72 (8.4045, 6.1341) -> (8.4045, 6.0579) centre (8.4045, 6.096) ccw
  line L35 (10.668, 6.096) -> (12.763, 6.096)
  arc A73 (12.763, 6.0579) -> (12.763, 6.1341) centre (12.763, 6.096) ccw
  arc A74 (10.668, 6.1341) -> (10.668, 6.0579) centre (10.668, 6.096) ccw
  line L36 (8.7493, 5.9436) -> (10.4902, 5.9436)
  arc A75 (10.4902, 5.9055) -> (10.4902, 5.9817) centre (10.4902, 5.9436) ccw
  arc A76 (8.7493, 5.9817) -> (8.7493, 5.9055) centre (8.7493, 5.9436) ccw
  line L37 (10.668, 5.9436) -> (12.4074, 5.9436)
  arc A77 (12.4074, 5.9055) -> (12.4074, 5.9817) centre (12.4074, 5.9436) ccw
  arc A78 (10.668, 5.9817) -> (10.668, 5.9055) centre (10.668, 5.9436) ccw
  line L38 (9.1733, 5.7912) -> (10.4902, 5.7912)
  arc A79 (10.4902, 5.7531) -> (10.4902, 5.8293) centre (10.4902, 5.7912) ccw
  arc A80 (9.1733, 5.8293) -> (9.1733, 5.7531) centre (9.1733, 5.7912) ccw
  line L39 (10.668, 5.7912) -> (11.9796, 5.7912)
  arc A81 (11.9796, 5.7531) -> (11.9796, 5.8293) centre (11.9796, 5.7912) ccw
  arc A82 (10.668, 5.8293) -> (10.668, 5.7531) centre (10.668, 5.7912) ccw
  line L40 (9.8815, 5.6388) -> (10.4902, 5.6388)
  arc A83 (10.4902, 5.6007) -> (10.4902, 5.6769) centre (10.4902, 5.6388) ccw
  arc A84 (9.8815, 5.6769) -> (9.8815, 5.6007) centre (9.8815, 5.6388) ccw
  line L41 (10.668, 5.6388) -> (11.2376, 5.6388)
  arc A85 (11.2376, 5.6007) -> (11.2376, 5.6769) centre (11.2376, 5.6388) ccw
  arc A86 (10.668, 5.6769) -> (10.668, 5.6007) centre (10.668, 5.6388) ccw
  line L42 (16.002, 15.494) -> (16.002, 14.986)
  arc A87 (15.9385, 14.986) -> (16.0655, 14.986) centre (16.002, 14.986) ccw
  arc A88 (16.0655, 15.494) -> (15.9385, 15.494) centre (16.002, 15.494) ccw
  line L43 (16.002, 14.986) -> (17.78, 13.208)
  arc A89 (17.7351, 13.1631) -> (17.8249, 13.2529) centre (17.78, 13.208) ccw
  arc A90 (16.0469, 15.0309) -> (15.9571, 14.9411) centre (16.002, 14.986) ccw
  line L44 (4.064, 31.242) -> (4.064, 21.336)
  arc A91 (4.0005, 21.336) -> (4.1275, 21.336) centre (4.064, 21.336) ccw
  arc A92 (4.1275, 31.242) -> (4.0005, 31.242) centre (4.064, 31.242) ccw
  line L45 (4.064, 21.336) -> (8.128, 17.272)
  arc A93 (8.0831, 17.2271) -> (8.1729, 17.3169) centre (8.128, 17.272) ccw
  arc A94 (4.1089, 21.3809) -> (4.0191, 21.2911) centre (4.064, 21.336) ccw
  line L46 (8.128, 17.272) -> (11.6876, 17.272)
  arc A95 (11.6876, 17.2085) -> (11.6876, 17.3355) centre (11.6876, 17.272) ccw
  arc A96 (8.128, 17.3355) -> (8.128, 17.2085) centre (8.128, 17.272) ccw
  line L47 (11.6876, 17.272) -> (12.2461, 17.8305)
  arc A97 (12.291, 17.7856) -> (12.2011, 17.8754) centre (12.2461, 17.8305) ccw
  arc A98 (11.6427, 17.3169) -> (11.7325, 17.2271) centre (11.6876, 17.272) ccw
  line L48 (33.528, 17.78) -> (30.099, 17.78)
  arc A99 (30.099, 17.8435) -> (30.099, 17.7165) centre (30.099, 17.78) ccw
  arc A100 (33.528, 17.7165) -> (33.528, 17.8435) centre (33.528, 17.78) ccw
  line L49 (30.099, 17.78) -> (26.6065, 21.2725)
  arc A101 (26.6514, 21.3174) -> (26.5616, 21.2276) centre (26.6065, 21.2725) ccw
  arc A102 (30.0541, 17.7351) -> (30.1439, 17.8249) centre (30.099, 17.78) ccw
  line L50 (26.6065, 21.2725) -> (26.162, 21.717)
  arc A103 (26.2069, 21.7619) -> (26.1171, 21.6721) centre (26.162, 21.717) ccw
  arc A104 (26.5616, 21.2276) -> (26.6514, 21.3174) centre (26.6065, 21.2725) ccw
  line L51 (30.4386, 33.657) -> (30.6027, 33.1762)
  arc A105 (30.5392, 33.1762) -> (30.6662, 33.1762) centre (30.6027, 33.1762) ccw
  arc A106 (30.5021, 33.657) -> (30.3751, 33.657) centre (30.4386, 33.657) ccw
  line L52 (30.6027, 33.1762) -> (28.702, 29.3074)
  arc A107 (28.6571, 29.3523) -> (28.7469, 29.2625) centre (28.702, 29.3074) ccw
  arc A108 (30.6476, 33.1313) -> (30.5578, 33.2211) centre (30.6027, 33.1762) ccw
  line L53 (28.702, 29.3074) -> (28.702, 29.718)
  arc A109 (28.6385, 29.718) -> (28.7655, 29.718) centre (28.702, 29.718) ccw
  arc A110 (28.7523, 29.3462) -> (28.6517, 29.2686) centre (28.702, 29.3074) ccw
  line L54 (28.702, 29.718) -> (29.972, 28.448)
  arc A111 (29.9271, 28.4031) -> (30.0169, 28.4929) centre (29.972, 28.448) ccw
  arc A112 (28.7469, 29.7629) -> (28.6571, 29.6731) centre (28.702, 29.718) ccw
  line L55 (29.972, 28.448) -> (29.972, 24.638)
  arc A113 (29.9085, 24.638) -> (30.0355, 24.638) centre (29.972, 24.638) ccw
  arc A114 (30.0355, 28.448) -> (29.9085, 28.448) centre (29.972, 28.448) ccw
  line L56 (29.972, 24.638) -> (26.6065, 21.2725)
  arc A115 (26.5616, 21.3174) -> (26.6514, 21.2276) centre (26.6065, 21.2725) ccw
  arc A116 (30.0169, 24.5931) -> (29.9271, 24.6829) centre (29.972, 24.638) ccw
  line L57 (9.4059, 20.2985) -> (10.668, 21.5763)
  arc A117 (10.7129, 21.5314) -> (10.6231, 21.6212) centre (10.668, 21.5763) ccw
  arc A118 (9.361, 20.3434) -> (9.4508, 20.2535) centre (9.4059, 20.2985) ccw
  line L58 (10.668, 21.5763) -> (12.7006, 21.6016)
  arc A119 (12.7006, 21.5381) -> (12.7006, 21.6651) centre (12.7006, 21.6016) ccw
  arc A120 (10.668, 21.6398) -> (10.668, 21.5128) centre (10.668, 21.5763) ccw
  line L59 (12.7006, 21.6016) -> (14.4564, 23.4016)
  arc A121 (14.5013, 23.3567) -> (14.4115, 23.4465) centre (14.4564, 23.4016) ccw
  arc A122 (12.6557, 21.6465) -> (12.7455, 21.5567) centre (12.7006, 21.6016) ccw
  line L60 (14.4564, 23.4016) -> (8.299, 31.8641)
  arc A123 (8.3625, 31.8641) -> (8.2355, 31.8641) centre (8.299, 31.8641) ccw
  arc A124 (14.3929, 23.4016) -> (14.5199, 23.4016) centre (14.4564, 23.4016) ccw
  line L61 (8.299, 31.8641) -> (8.4389, 32.7512)
  arc A125 (8.4838, 32.7063) -> (8.3761, 32.7611) centre (8.4389, 32.7512) ccw
  arc A126 (8.2541, 31.9091) -> (8.3439, 31.8192) centre (8.299, 31.8641) ccw
  line L62 (18.6224, 48.3279) -> (17.8752, 49.3548)
  arc A127 (17.9387, 49.3548) -> (17.8117, 49.3548) centre (17.8752, 49.3548) ccw
  arc A128 (18.5589, 48.3279) -> (18.6859, 48.3279) centre (18.6224, 48.3279) ccw
  line L63 (17.8752, 49.3548) -> (16.1011, 49.6346)
  arc A129 (16.146, 49.6795) -> (16.0562, 49.5897) centre (16.1011, 49.6346) ccw
  arc A130 (17.8303, 49.3099) -> (17.9201, 49.3997) centre (17.8752, 49.3548) ccw
  line L64 (16.1011, 49.6346) -> (11.5826, 46.3469)
  arc A131 (11.5826, 46.4104) -> (11.5826, 46.2834) centre (11.5826, 46.3469) ccw
  arc A132 (16.1011, 49.5711) -> (16.1011, 49.6981) centre (16.1011, 49.6346) ccw
  line L65 (11.5826, 46.3469) -> (10.5196, 39.6052)
  arc A133 (10.4747, 39.6501) -> (10.5645, 39.5603) centre (10.5196, 39.6052) ccw
  arc A134 (11.6275, 46.302) -> (11.5377, 46.3918) centre (11.5826, 46.3469) ccw
  line L66 (10.5196, 39.6052) -> (7.4388, 37.3636)
  arc A135 (7.4388, 37.4271) -> (7.4388, 37.3001) centre (7.4388, 37.3636) ccw
  arc A136 (10.5196, 39.5417) -> (10.5196, 39.6687) centre (10.5196, 39.6052) ccw
  line L67 (7.4388, 37.3636) -> (4.955, 37.7552)
  arc A137 (4.9999, 37.8001) -> (4.9101, 37.7103) centre (4.955, 37.7552) ccw
  arc A138 (7.3939, 37.3187) -> (7.4837, 37.4085) centre (7.4388, 37.3636) ccw
  line L68 (4.955, 37.7552) -> (3.5173, 36.7091)
  arc A139 (3.5173, 36.7726) -> (3.5173, 36.6456) centre (3.5173, 36.7091) ccw
  arc A140 (4.955, 37.6917) -> (4.955, 37.8187) centre (4.955, 37.7552) ccw
  line L69 (3.5173, 36.7091) -> (3.1257, 34.2254)
  arc A141 (3.0807, 34.2703) -> (3.1706, 34.1804) centre (3.1257, 34.2254) ccw
  arc A142 (3.5622, 36.6642) -> (3.4724, 36.754) centre (3.5173, 36.7091) ccw
  line L70 (3.1257, 34.2254) -> (4.2461, 34.4123)
  arc A143 (4.2177, 34.3555) -> (4.2745, 34.4691) centre (4.2461, 34.4123) ccw
  arc A144 (3.1541, 34.2821) -> (3.0973, 34.1686) centre (3.1257, 34.2254) ccw
  line L71 (4.2461, 34.4123) -> (7.4395, 33.9088)
  arc A145 (7.3946, 33.8639) -> (7.4844, 33.9537) centre (7.4395, 33.9088) ccw
  arc A146 (4.291, 34.4572) -> (4.2012, 34.3674) centre (4.2461, 34.4123) ccw
  line L72 (7.4395, 33.9088) -> (8.2614, 32.7792)
  arc A147 (8.1979, 32.7792) -> (8.3249, 32.7792) centre (8.2614, 32.7792) ccw
  arc A148 (7.503, 33.9088) -> (7.376, 33.9088) centre (7.4395, 33.9088) ccw
  line L73 (8.2614, 32.7792) -> (8.4389, 32.7512)
  arc A149 (8.429, 32.6885) -> (8.4838, 32.7961) centre (8.4389, 32.7512) ccw
  arc A150 (8.3063, 32.8241) -> (8.2165, 32.7343) centre (8.2614, 32.7792) ccw
  line L74 (20.828, 15.494) -> (20.828, 11.557)
  arc A151 (20.7645, 11.557) -> (20.8915, 11.557) centre (20.828, 11.557) ccw
  arc A152 (20.8915, 15.494) -> (20.7645, 15.494) centre (20.828, 15.494) ccw
  line L75 (20.828, 11.557) -> (21.717, 10.668)
  arc A153 (21.6721, 10.6231) -> (21.7619, 10.7129) centre (21.717, 10.668) ccw
  arc A154 (20.8729, 11.6019) -> (20.7831, 11.5121) centre (20.828, 11.557) ccw
  line L76 (35.5598, 28.194) -> (35.5599, 15.24)
  arc A155 (35.4964, 15.24) -> (35.6234, 15.24) centre (35.5599, 15.24) ccw
  arc A156 (35.6233, 28.194) -> (35.4963, 28.194) centre (35.5598, 28.194) ccw
  line L77 (35.5599, 15.24) -> (30.734, 10.414)
  arc A157 (30.6891, 10.4589) -> (30.7789, 10.3691) centre (30.734, 10.414) ccw
  arc A158 (35.6048, 15.1951) -> (35.515, 15.2849) centre (35.5599, 15.24) ccw
  line L78 (30.734, 10.414) -> (30.734, 9.398)
  arc A159 (30.6705, 9.398) -> (30.7975, 9.398) centre (30.734, 9.398) ccw
  arc A160 (30.7975, 10.414) -> (30.6705, 10.414) centre (30.734, 10.414) ccw
  line L79 (30.734, 9.398) -> (27.686, 6.35)
  arc A161 (27.6411, 6.3949) -> (27.7309, 6.3051) centre (27.686, 6.35) ccw
  arc A162 (30.7789, 9.3531) -> (30.6891, 9.4429) centre (30.734, 9.398) ccw
  line L80 (27.686, 6.35) -> (24.384, 6.35)
  arc A163 (24.384, 6.4135) -> (24.384, 6.2865) centre (24.384, 6.35) ccw
  arc A164 (27.686, 6.2865) -> (27.686, 6.4135) centre (27.686, 6.35) ccw
  line L81 (24.384, 6.35) -> (22.352, 8.382)
  arc A165 (22.3969, 8.4269) -> (22.3071, 8.3371) centre (22.352, 8.382) ccw
  arc A166 (24.3391, 6.3051) -> (24.4289, 6.3949) centre (24.384, 6.35) ccw
  line L82 (22.352, 8.382) -> (22.352, 10.033)
  arc A167 (22.4155, 10.033) -> (22.2885, 10.033) centre (22.352, 10.033) ccw
  arc A168 (22.2885, 8.382) -> (22.4155, 8.382) centre (22.352, 8.382) ccw
  line L83 (22.352, 10.033) -> (21.717, 10.668)
  arc A169 (21.7619, 10.7129) -> (21.6721, 10.6231) centre (21.717, 10.668) ccw
  arc A170 (22.3071, 9.9881) -> (22.3969, 10.0779) centre (22.352, 10.033) ccw
  line L84 (34.29, 16.256) -> (28.194, 16.256)
  arc A171 (28.194, 16.3195) -> (28.194, 16.1925) centre (28.194, 16.256) ccw
  arc A172 (34.29, 16.1925) -> (34.29, 16.3195) centre (34.29, 16.256) ccw
  line L85 (28.194, 16.256) -> (27.94, 16.51)
  arc A173 (27.9849, 16.5549) -> (27.8951, 16.4651) centre (27.94, 16.51) ccw
  arc A174 (28.1491, 16.2111) -> (28.2389, 16.3009) centre (28.194, 16.256) ccw
  line L86 (27.94, 16.51) -> (14.732, 16.51)
  arc A175 (14.732, 16.5735) -> (14.732, 16.4465) centre (14.732, 16.51) ccw
  arc A176 (27.94, 16.4465) -> (27.94, 16.5735) centre (27.94, 16.51) ccw
  line L87 (12.446, 16.51) -> (12.065, 16.51)
  arc A177 (12.065, 16.5735) -> (12.065, 16.4465) centre (12.065, 16.51) ccw
  arc A178 (12.446, 16.4465) -> (12.446, 16.5735) centre (12.446, 16.51) ccw
  line L88 (12.065, 16.51) -> (10.668, 15.113)
  arc A179 (10.6231, 15.1579) -> (10.7129, 15.0681) centre (10.668, 15.113) ccw
  arc A180 (12.1099, 16.4651) -> (12.0201, 16.5549) centre (12.065, 16.51) ccw
  line L89 (14.732, 16.51) -> (12.446, 16.51)
  arc A181 (12.446, 16.5735) -> (12.446, 16.4465) centre (12.446, 16.51) ccw
  arc A182 (14.732, 16.4465) -> (14.732, 16.5735) centre (14.732, 16.51) ccw
  line L90 (-1.016, -0.762) -> (37.592, -0.762)
  arc A183 (37.592, -0.8636) -> (37.592, -0.6604) centre (37.592, -0.762) ccw
  arc A184 (-1.016, -0.6604) -> (-1.016, -0.8636) centre (-1.016, -0.762) ccw
  line L91 (37.592, -0.762) -> (37.338, 37.846)
  arc A185 (37.4396, 37.8467) -> (37.2364, 37.8453) centre (37.338, 37.846) ccw
  arc A186 (37.4904, -0.7627) -> (37.6936, -0.7613) centre (37.592, -0.762) ccw
  line L92 (37.338, 37.846) -> (27.94, 37.846)
  arc A187 (27.94, 37.9476) -> (27.94, 37.7444) centre (27.94, 37.846) ccw
  arc A188 (37.338, 37.7444) -> (37.338, 37.9476) centre (37.338, 37.846) ccw
  line L93 (27.94, 37.846) -> (27.94, 34.29)
  arc A189 (27.8384, 34.29) -> (28.0416, 34.29) centre (27.94, 34.29) ccw
  arc A190 (28.0416, 37.846) -> (27.8384, 37.846) centre (27.94, 37.846) ccw
  line L94 (27.94, 34.29) -> (27.686, 34.036)
  arc A191 (27.6142, 34.1078) -> (27.7578, 33.9642) centre (27.686, 34.036) ccw
  arc A192 (28.0118, 34.2182) -> (27.8682, 34.3618) centre (27.94, 34.29) ccw
  line L95 (27.686, 34.036) -> (25.654, 34.036)
  arc A193 (25.654, 34.1376) -> (25.654, 33.9344) centre (25.654, 34.036) ccw
  arc A194 (27.686, 33.9344) -> (27.686, 34.1376) centre (27.686, 34.036) ccw
  line L96 (25.654, 34.036) -> (21.336, 29.718)
  arc A195 (21.2642, 29.7898) -> (21.4078, 29.6462) centre (21.336, 29.718) ccw
  arc A196 (25.7258, 33.9642) -> (25.5822, 34.1078) centre (25.654, 34.036) ccw
  line L97 (21.336, 29.718) -> (18.542, 32.512)
  arc A197 (18.6138, 32.5838) -> (18.4702, 32.4402) centre (18.542, 32.512) ccw